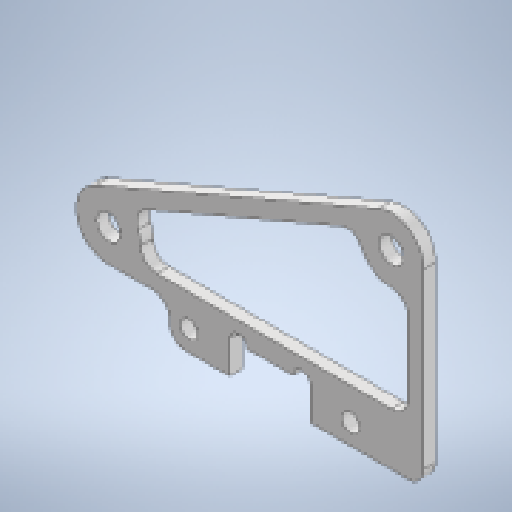
# Autodesk Inventor part: シン・足首
Saved by Autodesk Inventor 2024 (Build 280153000, 153)
## iProperties
Created: 2023-11-03
Part Number: シン・足首
Material: 一般
Document SubType Name: Modeling
Designer: right
Density: 1 g/cm^3
Appearance: 既定
Author: right
Autodesk Inventor part; units mm, degrees
ref_plane "YZ Plane" through (0, 0, 0) normal (1, 0, 0) x (0, 1, 0)
ref_plane "XZ Plane" through (0, 0, 0) normal (0, 1, 0) x (-1, 0, 0)
ref_plane "XY Plane" through (0, 0, 0) normal (0, 0, 1) x (1, 0, 0)
sketch "スケッチ1" plane through (0, 0, 0) normal (0, 0, 1) x (1, 0, 0)
  circle A0 centre (-17.5, -7.5) radius 1.5
  circle A1 centre (17.5, 7.5) radius 1.5
  circle A2 centre (-17.5, -7.5) radius 4
  circle A3 centre (17.5, 7.5) radius 4
  line L0 (-2.5, -12.5) -> (7.5, -12.5)
  line L1 (7.5, -12.5) -> (7.5, -15.5)
  line L2 (7.5, -15.5) -> (-2.5, -15.5)
  line L3 (-2.5, -15.5) -> (-2.5, -12.5)
  circle A4 centre (-1.4, -12.5) radius 1.1
  line L4 (-2.5, -14) -> (7.5, -14) construction
  line L5 (2.5, -14) -> (2.5, -12.5) construction
  circle A5 centre (-1.4, -15.5) radius 1.1
  circle A6 centre (6.4, -12.5) radius 1.1
  circle A7 centre (6.4, -15.5) radius 1.1
  circle A8 centre (-7.5, -14) radius 1.1
  circle A9 centre (12.5, -14) radius 1.1
  line L6 (-19.0757, -3.8234) -> (15.9243, 11.1766)
  line L7 (21.5, 7.5) -> (21.5, -11.5)
  line L8 (-10, -11.5) -> (21.5, -11.5)
  line L9 (21.5, -11.5) -> (21.5, -16.5)
  line L10 (21.5, -16.5) -> (-10, -16.5)
  line L11 (-10, -16.5) -> (-10, -11.5)
  line L12 (-2.5, -15.5) -> (-2.5, -16.5)
  line L13 (7.5, -15.5) -> (7.5, -16.5)
  line L14 (-17.5, -11.5) -> (-10, -11.5)
  line L15 (21.5, -11.5) -> (21.5, -11.5)
  line L16 (-14.0359, -9.5) -> (19.5, -9.5)
  line L17 (19.5, 4.0359) -> (19.5, -9.5)
  line L18 (-15.1038, -4.2971) -> (13.5281, 7.9737)
  point P0 (0, 0)
  point P1 (-0.3, -12.5)
  point P2 (5.3, -12.5)
  point P3 (7.5, -12.5)
  dimension "d12" = 2.2
  dimension "d0" = 3
  dimension "d1" = 3
  dimension "d2" = 35
  dimension "d5" = 7.5
  dimension "d6" = 15
  dimension "d7" = 17.5
  dimension "d8" = 8
  dimension "d9" = 8
  dimension "d10" = 10
  dimension "d11" = 3
  dimension "d13" = 2.2
  dimension "d14" = 5
  dimension "d15" = 20
  dimension "d19" = 2.5
  dimension "d21" = 1
  dimension "d22" = 2
  dimension "d23" = 2
  dimension "d24" = 2
  dimension "d29" = 5
  constraints: 39 end point, 9 centre point, 8 point on circle, 6 parallel, 6 perpendicular, 6 tangent, 5 point on line, 4 coincident, 4 midpoint, 4 symmetric about line, 3 horizontal, 2 horizontal alignment, 2 vertical, 7 other
  measures "d0" diameter of A0
  measures "d1" diameter of A1
  measures "d2" horizontal distance of A1.centre A0.centre
  measures "d5" vertical distance of A1.centre point (0, 0)
  measures "d6" vertical distance of A1.centre A0.centre
  measures "d7" horizontal distance of point (0, 0) A0.centre
  measures "d8" diameter of A2
  measures "d9" diameter of A3
  measures "d10" distance of L1.end L2.end
  measures "d11" distance of L0.end L1.end
  measures "d13" diameter of A8
  measures "d14" distance from line of L3 A8.centre
  measures "d15" horizontal distance of L5.start A0.centre
  measures "d19" distance from line of L11 A8.centre
  measures "d21" distance between parallel lines of L10 L2
  measures "d22" distance between parallel lines of L8 L16
  measures "d23" distance between parallel lines of L7 L17
  measures "d24" distance between parallel lines of L6 L18
  measures "d29" distance between parallel lines of L8 L10
extrude "押し出し1" add sketch "スケッチ1" along normal blind 1.5 contours A2 | A2 L6 A3 L18 | L16 L17 A3 L7 L8 A6 A4 L14 A2 | A3 | L8 A4 L3 L12 L10 L11 | L9 L10 L13 L1 A6 L8 | L8 A6 L0 A4
fillet "フィレット1" radius 2 8 edges at (-10, -16.5, 0.75) (-10, -11.5, 0.75) (19.5, -9.5, 0.75) (21.5, -16.5, 0.75) (19.5, 4.0359, 0.75) (13.5281, 7.9737, 0.75) (-14.0359, -9.5, 0.75) (-15.1038, -4.2971, 0.75)
equation "\"d7\" = 0.5 * d2"
equation "\"d8\" = d9"
equation "\"d22\" = d24"
equation "\"d24\" = d23"
